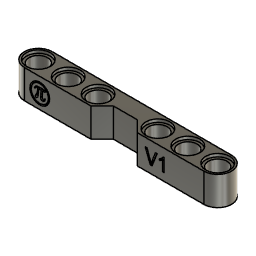
4. BLDC motor transmission 7x bar [V1] (Autodesk Fusion 360 design; units mm, degrees)
Autodesk Fusion 360 part; units mm, degrees
note: some values were not read from the file. Set by a fixed rule: which sketch regions a step uses.
sketch "Base" plane through (0, 0, 0) normal (0, 0, 1) x (1, 0, 0)
  line L0 (3.7, 0) -> (51.7, 0)
  line L1 (51.7, 7.4) -> (3.7, 7.4)
  line L2 (27.7, 7.4) -> (27.7, 0)
  line L3 (0, 3.7) -> (55.4, 3.7)
  circle A0 centre (27.7, 3.7) radius 2.5
  circle A1 centre (27.7, 3.7) radius 3.2
  circle A2 centre (35.7, 3.7) radius 3.2
  circle A3 centre (35.7, 3.7) radius 2.5
  circle A4 centre (43.7, 3.7) radius 3.2
  circle A5 centre (43.7, 3.7) radius 2.5
  circle A6 centre (51.7, 3.7) radius 3.2
  circle A7 centre (51.7, 3.7) radius 2.5
  circle A8 centre (19.7, 3.7) radius 2.5
  circle A9 centre (19.7, 3.7) radius 3.2
  circle A10 centre (11.7, 3.7) radius 2.5
  circle A11 centre (11.7, 3.7) radius 3.2
  circle A12 centre (3.7, 3.7) radius 2.5
  circle A13 centre (3.7, 3.7) radius 3.2
  arc A14 (3.7, 7.4) -> (0, 3.7) centre (3.7, 3.7) ccw
  arc A15 (0, 3.7) -> (3.7, 0) centre (3.7, 3.7) ccw
  arc A16 (55.4, 3.7) -> (51.7, 7.4) centre (51.7, 3.7) ccw
  arc A17 (51.7, 0) -> (55.4, 3.7) centre (51.7, 3.7) ccw
  line L4 (21.5, 0) -> (24.5, 3)
  line L5 (21.5, 0) -> (25.7426, 0) construction
  line L6 (24.5, 3) -> (30.9, 3)
  line L7 (30.9, 3) -> (33.9, 0)
  point P0 (55.4, 0)
  point P1 (0, 7.4)
  dimension "d1" = 55.4
  dimension "d2" = 7.4
  dimension "d3" = 5
  dimension "d4" = 6.4
  dimension "d7" = 24
  dimension "d8" = 0
  dimension "d11" = -24
  dimension "d12" = 0
  dimension "d13" = 3.7
  dimension "d14" = 3.7
  dimension "d15" = 3.7
  dimension "d16" = 3.7
  dimension "d17" = 45
  dimension "d18" = 135
  constraint horizontal L0
  constraint horizontal L1
  constraint midpoint L3 A0.centre
  constraint concentric A0 A1
  constraint coincident L1 L2.start
  constraint coincident P1 L1
  constraint tangent L1 A14
  constraint coincident L0 L2.end
  constraint coincident origin L0
  constraint tangent L0 A15
  constraint coincident L3.start A14.end
  constraint tangent L1 A16
  constraint coincident P0 L0
  constraint tangent L0 A17
  constraint coincident L3.end A16.start
  constraint horizontal L5
  constraint coincident L0 L4.start
  constraint perpendicular L2 L6
  constraint coincident L0 L7.end
  measures "d1" distance of origin P0
  measures "d2" distance of origin P1
  measures "d3" diameter of A0
  measures "d4" diameter of A1
  measures "d13" radius of A14
  measures "d14" radius of A15
  measures "d15" radius of A16
  measures "d16" radius of A17
  measures "d17" angle of L4 L5
  measures "d18" angle of L6 L7
extrude "Extrude1" add sketch "Base" along normal blind 7.7 contours L0 L3 A1 A9 A11 A13 A15 L4 L6 | L1 L2 L3 A1 A9 A11 A13 A14 | L0 L3 A1 A2 A4 A6 A17 L6 L7 | L3 A0 A1 L6 | L1 L2 L3 A1 A2 A4 A6 A16 | L3 A0 A1 L6 | L2 L3 A0 A1 | L2 L3 A0 L6 | L2 L3 A0 A1 | L2 L3 A0 L6 | L2 L3 A0 | L2 L3 A0
extrude "Extrude3" add sketch "Base" along normal blind 6.9 contours L3 A12 A13 | L3 A12 A13 | L3 A10 A11 | L3 A10 A11 | L3 A8 A9 | L3 A8 A9 | L3 A6 A7 | L3 A6 A7 | L3 A2 A3 | L3 A2 A3 | L3 A4 A5 | L3 A4 A5
extrude "Extrude4" cut sketch "Base" along normal blind 0.8 contours L3 A12 A13 | L3 A12 A13 | L3 A10 A11 | L3 A10 A11 | L3 A8 A9 | L3 A8 A9 | L3 A6 A7 | L3 A6 A7 | L3 A2 A3 | L3 A2 A3 | L3 A4 A5 | L3 A4 A5
sketch "Author" plane through (0, 0, 0) normal (0, -1, 0) x (1, 0, 0)
  line L0 (3.7, 0) -> (21.5, 0)
  line L1 (21.5, 0) -> (21.5, 7.7)
  line L2 (21.5, 7.7) -> (3.7, 7.7)
  line L3 (3.7, 7.7) -> (3.7, 0)
  line L4 (6.3372, 4.2854) -> (6.4432, 4.2775)
  spline S0 degree 3 poles (6.4432, 4.2775) (6.5532, 4.4019) (6.5964, 4.7698) (7.2445, 4.6978) knots 0 0 0 0 1 1 1 1
  spline S1 degree 3 poles (7.2445, 4.6978) (7.2209, 3.1215) (6.5296, 2.9552) (6.5728, 2.6318) knots 0 0 0 0 1 1 1 1
  spline S2 degree 3 poles (6.5728, 2.6318) (6.5885, 2.4485) (6.7339, 2.3359) (6.891, 2.3294) knots 0 0 0 0 1 1 1 1
  spline S3 degree 3 poles (6.891, 2.3294) (7.3872, 2.3464) (7.3649, 3.0154) (7.5194, 4.7017) knots 0 0 0 0 1 1 1 1
  line L5 (7.5194, 4.7017) -> (8.1596, 4.7017)
  spline S4 degree 3 poles (8.1596, 4.7017) (8.1256, 4.1073) (8.0326, 3.5129) (8.0222, 2.9303) knots 0 0 0 0 1 1 1 1
  spline S5 degree 3 poles (8.0222, 2.9303) (8.03, 2.5428) (8.2657, 2.3359) (8.576, 2.3333) knots 0 0 0 0 1 1 1 1
  spline S6 degree 3 poles (8.576, 2.3333) (9.0866, 2.3163) (9.2476, 2.912) (9.2476, 3.166) knots 0 0 0 0 1 1 1 1
  line L6 (9.2476, 3.166) -> (9.1376, 3.166)
  spline S7 degree 3 poles (9.1376, 3.166) (9.1271, 2.9565) (9.0263, 2.8059) (8.8116, 2.7968) knots 0 0 0 0 1 1 1 1
  spline S8 degree 3 poles (8.8116, 2.7968) (8.2264, 2.7889) (8.5485, 3.8258) (8.5524, 4.6938) knots 0 0 0 0 1 1 1 1
  line L7 (8.5524, 4.6938) -> (9.2476, 4.6899)
  line L8 (9.2476, 4.6899) -> (9.2437, 5.1337)
  spline S9 degree 3 poles (9.2437, 5.1337) (6.3541, 5.1477) (6.7209, 5.2044) (6.3372, 4.2854) knots 0 0 0 0 1 1 1 1
  arc A0 (5.1466, 3.7345) -> (7.7924, 6.3803) centre (7.7924, 3.7345) cw
  arc A1 (7.7924, 1.0887) -> (5.1466, 3.7345) centre (7.7924, 3.7345) cw
  arc A2 (10.4382, 3.7345) -> (7.7924, 1.0887) centre (7.7924, 3.7345) cw
  arc A3 (7.7924, 6.3803) -> (10.4382, 3.7345) centre (7.7924, 3.7345) cw
  arc A4 (7.7924, 6.0264) -> (7.8514, 6.0256) centre (7.7927, 3.7345) cw
  arc A5 (7.8514, 6.0256) -> (7.9104, 6.0233) centre (7.7922, 3.7345) cw
  arc A6 (7.9104, 6.0233) -> (7.9693, 6.0195) centre (7.7922, 3.7345) cw
  arc A7 (7.9693, 6.0195) -> (8.028, 6.0142) centre (7.7927, 3.7345) cw
  arc A8 (8.028, 6.0142) -> (8.0867, 6.0074) centre (7.7924, 3.7345) cw
  arc A9 (8.0867, 6.0074) -> (8.1451, 5.9991) centre (7.7925, 3.7345) cw
  arc A10 (8.1451, 5.9991) -> (8.2033, 5.9892) centre (7.7919, 3.7346) cw
  arc A11 (8.2033, 5.9892) -> (8.2612, 5.9779) centre (7.7926, 3.7344) cw
  arc A12 (8.2612, 5.9779) -> (8.3188, 5.9651) centre (7.7926, 3.7344) cw
  arc A13 (8.3188, 5.9651) -> (8.3761, 5.9508) centre (7.792, 3.7346) cw
  arc A14 (8.3761, 5.9508) -> (8.4329, 5.935) centre (7.7929, 3.7343) cw
  arc A15 (8.4329, 5.935) -> (8.4894, 5.9178) centre (7.7921, 3.7346) cw
  arc A16 (8.4894, 5.9178) -> (8.5454, 5.8991) centre (7.7922, 3.7345) cw
  arc A17 (8.5454, 5.8991) -> (8.6008, 5.879) centre (7.7926, 3.7344) cw
  arc A18 (8.6008, 5.879) -> (8.6558, 5.8575) centre (7.7922, 3.7346) cw
  arc A19 (8.6558, 5.8575) -> (8.7102, 5.8346) centre (7.7926, 3.7344) cw
  arc A20 (8.7102, 5.8346) -> (8.7639, 5.8102) centre (7.7926, 3.7344) cw
  arc A21 (8.7639, 5.8102) -> (8.8171, 5.7845) centre (7.7923, 3.7345) cw
  arc A22 (8.8171, 5.7845) -> (8.8695, 5.7575) centre (7.7926, 3.7344) cw
  arc A23 (8.8695, 5.7575) -> (8.9212, 5.7291) centre (7.792, 3.7347) cw
  arc A24 (8.9212, 5.7291) -> (8.9722, 5.6993) centre (7.7925, 3.7344) cw
  arc A25 (8.9722, 5.6993) -> (9.0224, 5.6683) centre (7.7923, 3.7345) cw
  arc A26 (9.0224, 5.6683) -> (9.0718, 5.636) centre (7.7923, 3.7346) cw
  arc A27 (9.0718, 5.636) -> (9.1203, 5.6024) centre (7.7926, 3.7343) cw
  arc A28 (9.1203, 5.6024) -> (9.168, 5.5676) centre (7.7925, 3.7344) cw
  arc A29 (9.168, 5.5676) -> (9.2147, 5.5316) centre (7.7922, 3.7346) cw
  arc A30 (9.2147, 5.5316) -> (9.2605, 5.4944) centre (7.7925, 3.7344) cw
  arc A31 (9.2605, 5.4944) -> (9.3054, 5.456) centre (7.7923, 3.7345) cw
  arc A32 (9.3054, 5.456) -> (9.3492, 5.4165) centre (7.7923, 3.7345) cw
  arc A33 (9.3492, 5.4165) -> (9.392, 5.3758) centre (7.7926, 3.7343) cw
  arc A34 (9.392, 5.3758) -> (9.4337, 5.3341) centre (7.7924, 3.7345) cw
  arc A35 (9.4337, 5.3341) -> (9.4744, 5.2913) centre (7.7922, 3.7347) cw
  arc A36 (9.4744, 5.2913) -> (9.5139, 5.2475) centre (7.7924, 3.7344) cw
  arc A37 (9.5139, 5.2475) -> (9.5523, 5.2026) centre (7.7924, 3.7344) cw
  arc A38 (9.5523, 5.2026) -> (9.5895, 5.1568) centre (7.7923, 3.7346) cw
  arc A39 (9.5895, 5.1568) -> (9.6255, 5.1101) centre (7.7925, 3.7343) cw
  arc A40 (9.6255, 5.1101) -> (9.6603, 5.0624) centre (7.7923, 3.7346) cw
  arc A41 (9.6603, 5.0624) -> (9.6939, 5.0139) centre (7.7922, 3.7347) cw
  arc A42 (9.6939, 5.0139) -> (9.7262, 4.9645) centre (7.7925, 3.7344) cw
  arc A43 (9.7262, 4.9645) -> (9.7572, 4.9143) centre (7.7924, 3.7344) cw
  arc A44 (9.7572, 4.9143) -> (9.787, 4.8633) centre (7.7923, 3.7346) cw
  arc A45 (9.787, 4.8633) -> (9.8154, 4.8116) centre (7.7926, 3.7341) cw
  arc A46 (9.8154, 4.8116) -> (9.8424, 4.7592) centre (7.7923, 3.7347) cw
  arc A47 (9.8424, 4.7592) -> (9.8681, 4.706) centre (7.7924, 3.7344) cw
  arc A48 (9.8681, 4.706) -> (9.8925, 4.6523) centre (7.7923, 3.7347) cw
  arc A49 (9.8925, 4.6523) -> (9.9154, 4.5979) centre (7.7925, 3.7342) cw
  arc A50 (9.9154, 4.5979) -> (9.9369, 4.5429) centre (7.7923, 3.7347) cw
  arc A51 (9.9369, 4.5429) -> (9.957, 4.4875) centre (7.7923, 3.7347) cw
  arc A52 (9.957, 4.4875) -> (9.9757, 4.4315) centre (7.7924, 3.7343) cw
  arc A53 (9.9757, 4.4315) -> (9.9929, 4.375) centre (7.7925, 3.7342) cw
  arc A54 (9.9929, 4.375) -> (10.0087, 4.3181) centre (7.7922, 3.735) cw
  arc A55 (10.0087, 4.3181) -> (10.023, 4.2609) centre (7.7925, 3.7341) cw
  arc A56 (10.023, 4.2609) -> (10.0358, 4.2033) centre (7.7923, 3.7347) cw
  arc A57 (10.0358, 4.2033) -> (10.0471, 4.1454) centre (7.7924, 3.7342) cw
  arc A58 (10.0471, 4.1454) -> (10.057, 4.0872) centre (7.7924, 3.7345) cw
  arc A59 (10.057, 4.0872) -> (10.0653, 4.0288) centre (7.7924, 3.7346) cw
  arc A60 (10.0653, 4.0288) -> (10.0721, 3.9701) centre (7.7924, 3.7345) cw
  arc A61 (10.0721, 3.9701) -> (10.0774, 3.9114) centre (7.7924, 3.7347) cw
  arc A62 (10.0774, 3.9114) -> (10.0812, 3.8525) centre (7.7924, 3.7343) cw
  arc A63 (10.0812, 3.8525) -> (10.0835, 3.7935) centre (7.7924, 3.7343) cw
  arc A64 (10.0835, 3.7935) -> (10.0843, 3.7345) centre (7.7924, 3.7348) cw
  arc A65 (10.0843, 3.7345) -> (10.0779, 3.5632) centre (7.7924, 3.7344) cw
  arc A66 (10.0779, 3.5632) -> (10.0587, 3.3929) centre (7.7924, 3.7346) cw
  arc A67 (10.0587, 3.3929) -> (10.0268, 3.2245) centre (7.7924, 3.7344) cw
  arc A68 (10.0268, 3.2245) -> (9.9824, 3.0589) centre (7.7924, 3.7345) cw
  arc A69 (9.9824, 3.0589) -> (9.9258, 2.8972) centre (7.7924, 3.7345) cw
  arc A70 (9.9258, 2.8972) -> (9.8573, 2.7401) centre (7.7924, 3.7345) cw
  arc A71 (9.8573, 2.7401) -> (9.7772, 2.5885) centre (7.7923, 3.7344) cw
  arc A72 (9.7772, 2.5885) -> (9.686, 2.4434) centre (7.7924, 3.7345) cw
  arc A73 (9.686, 2.4434) -> (9.5842, 2.3055) centre (7.7924, 3.7345) cw
  arc A74 (9.5842, 2.3055) -> (9.4724, 2.1756) centre (7.7924, 3.7345) cw
  arc A75 (9.4724, 2.1756) -> (9.3513, 2.0544) centre (7.7923, 3.7344) cw
  arc A76 (9.3513, 2.0544) -> (9.2213, 1.9426) centre (7.7925, 3.7346) cw
  arc A77 (9.2213, 1.9426) -> (9.0834, 1.8408) centre (7.7924, 3.7345) cw
  arc A78 (9.0834, 1.8408) -> (8.9383, 1.7497) centre (7.7924, 3.7345) cw
  arc A79 (8.9383, 1.7497) -> (8.7868, 1.6696) centre (7.7924, 3.7345) cw
  arc A80 (8.7868, 1.6696) -> (8.6297, 1.601) centre (7.7924, 3.7345) cw
  arc A81 (8.6297, 1.601) -> (8.4679, 1.5444) centre (7.7924, 3.7345) cw
  arc A82 (8.4679, 1.5444) -> (8.3024, 1.5001) centre (7.7923, 3.7345) cw
  arc A83 (8.3024, 1.5001) -> (8.134, 1.4682) centre (7.7924, 3.7345) cw
  arc A84 (8.134, 1.4682) -> (7.9637, 1.449) centre (7.7923, 3.7345) cw
  arc A85 (7.9637, 1.449) -> (7.7924, 1.4426) centre (7.7925, 3.7345) cw
  arc A86 (7.7924, 1.4426) -> (7.6211, 1.449) centre (7.7923, 3.7345) cw
  arc A87 (7.6211, 1.449) -> (7.4508, 1.4682) centre (7.7925, 3.7345) cw
  arc A88 (7.4508, 1.4682) -> (7.2824, 1.5001) centre (7.7923, 3.7345) cw
  arc A89 (7.2824, 1.5001) -> (7.1168, 1.5444) centre (7.7924, 3.7345) cw
  arc A90 (7.1168, 1.5444) -> (6.9551, 1.601) centre (7.7924, 3.7345) cw
  arc A91 (6.9551, 1.601) -> (6.798, 1.6696) centre (7.7924, 3.7345) cw
  arc A92 (6.798, 1.6696) -> (6.6464, 1.7497) centre (7.7924, 3.7345) cw
  arc A93 (6.6464, 1.7497) -> (6.5013, 1.8408) centre (7.7924, 3.7345) cw
  arc A94 (6.5013, 1.8408) -> (6.3634, 1.9426) centre (7.7924, 3.7345) cw
  arc A95 (6.3634, 1.9426) -> (6.2335, 2.0544) centre (7.7923, 3.7346) cw
  arc A96 (6.2335, 2.0544) -> (6.1123, 2.1756) centre (7.7924, 3.7345) cw
  arc A97 (6.1123, 2.1756) -> (6.0005, 2.3055) centre (7.7925, 3.7344) cw
  arc A98 (6.0005, 2.3055) -> (5.8987, 2.4434) centre (7.7924, 3.7345) cw
  arc A99 (5.8987, 2.4434) -> (5.8076, 2.5885) centre (7.7923, 3.7345) cw
  arc A100 (5.8076, 2.5885) -> (5.7275, 2.7401) centre (7.7924, 3.7344) cw
  arc A101 (5.7275, 2.7401) -> (5.6589, 2.8972) centre (7.7924, 3.7345) cw
  arc A102 (5.6589, 2.8972) -> (5.6023, 3.0589) centre (7.7924, 3.7345) cw
  arc A103 (5.6023, 3.0589) -> (5.558, 3.2245) centre (7.7924, 3.7345) cw
  arc A104 (5.558, 3.2245) -> (5.5261, 3.3929) centre (7.7924, 3.7344) cw
  arc A105 (5.5261, 3.3929) -> (5.5069, 3.5632) centre (7.7924, 3.7346) cw
  arc A106 (5.5069, 3.5632) -> (5.5005, 3.7345) centre (7.7924, 3.7344) cw
  arc A107 (5.5005, 3.7345) -> (5.5069, 3.9058) centre (7.7924, 3.7346) cw
  arc A108 (5.5069, 3.9058) -> (5.5261, 4.0761) centre (7.7924, 3.7344) cw
  arc A109 (5.5261, 4.0761) -> (5.558, 4.2445) centre (7.7924, 3.7346) cw
  arc A110 (5.558, 4.2445) -> (5.6023, 4.41) centre (7.7924, 3.7344) cw
  arc A111 (5.6023, 4.41) -> (5.6589, 4.5718) centre (7.7924, 3.7345) cw
  arc A112 (5.6589, 4.5718) -> (5.7275, 4.7289) centre (7.7924, 3.7345) cw
  arc A113 (5.7275, 4.7289) -> (5.8076, 4.8804) centre (7.7924, 3.7345) cw
  arc A114 (5.8076, 4.8804) -> (5.8987, 5.0255) centre (7.7924, 3.7345) cw
  arc A115 (5.8987, 5.0255) -> (6.0005, 5.1634) centre (7.7924, 3.7345) cw
  arc A116 (6.0005, 5.1634) -> (6.1123, 5.2934) centre (7.7925, 3.7346) cw
  arc A117 (6.1123, 5.2934) -> (6.2335, 5.4145) centre (7.7923, 3.7344) cw
  arc A118 (6.2335, 5.4145) -> (6.3634, 5.5263) centre (7.7924, 3.7345) cw
  arc A119 (6.3634, 5.5263) -> (6.5013, 5.6281) centre (7.7924, 3.7345) cw
  arc A120 (6.5013, 5.6281) -> (6.6464, 5.7193) centre (7.7924, 3.7345) cw
  arc A121 (6.6464, 5.7193) -> (6.798, 5.7994) centre (7.7924, 3.7345) cw
  arc A122 (6.798, 5.7994) -> (6.9551, 5.8679) centre (7.7924, 3.7345) cw
  arc A123 (6.9551, 5.8679) -> (7.1168, 5.9245) centre (7.7924, 3.7345) cw
  arc A124 (7.1168, 5.9245) -> (7.2824, 5.9689) centre (7.7924, 3.7345) cw
  arc A125 (7.2824, 5.9689) -> (7.4508, 6.0008) centre (7.7923, 3.7345) cw
  arc A126 (7.4508, 6.0008) -> (7.6211, 6.02) centre (7.7925, 3.7345) cw
  arc A127 (7.6211, 6.02) -> (7.7924, 6.0264) centre (7.7923, 3.7345) cw
sketch "Version" plane through (0, 0, 0) normal (0, -1, 0) x (1, 0, 0)
  line L0 (36, 2) -> (44, 2) construction
  line L1 (44, 2) -> (44, 6) construction
  line L2 (44, 6) -> (36, 6) construction
  line L3 (36, 6) -> (36, 2) construction
  dimension "d27" = 3.5
  text T0 "V1" font "Arial" height 3.5 align left bottom in box 8 x 4 at (36, 2) x (1, 0) y (0, 1) spacing 1
extrude "Extrude5" cut sketch "Author" sketch "Version" against normal blind 0.6 contours L4 S0 S1 S2 S3 L5 S4 S5 S6 L6 S7 S8 L7 L8 S9 | A0 A1 A2 A3 of sketch 2 text T0
named bodies: "Base"
